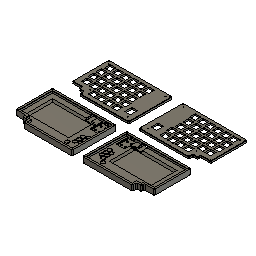
Split_Keyboardd (Autodesk Fusion 360 design; units mm, degrees)
part number: 2026-06-04-13-11-55-782
Autodesk Fusion 360 part; units mm, degrees
note: some values were not read from the file. Chosen so that the rebuilt part matches the saved one: which bodies a step acts on; which pieces of a blend or face edit are solid. Set by a fixed rule: which sketch regions a step uses; the direction of a hole.
(part 1 of 2)
sketch "Sketch1" plane through (0, 0, 0) normal (0, 1, 0) x (1, 0, 0)
  line L0 (174.75, 46) -> (174.75, -34.5)
  line L1 (174.75, -34.5) -> (149.75, -34.5)
  line L2 (149.75, -34.5) -> (149.75, -42)
  line L3 (149.75, -42) -> (138.25, -42)
  line L4 (138.25, -42) -> (138.25, -52.5)
  line L5 (138.25, -52.5) -> (24.5, -52.5)
  line L6 (25.5, 46) -> (24.5, -52.5)
  line L7 (-11.6355, 46.5) -> (-159.1355, 46.5)
  line L8 (-159.1355, 46.5) -> (-159.1355, -34)
  line L9 (-159.1355, -34) -> (-134.6355, -34)
  line L10 (-134.6355, -34) -> (-134.6355, -41.5)
  line L11 (-134.6355, -41.5) -> (-123.1355, -41.5)
  line L12 (-123.1355, -41.5) -> (-123.1355, -52)
  line L13 (-123.1355, -52) -> (-11.6355, -52)
  line L14 (-11.6355, -52) -> (-11.6355, 46.5)
  line L15 (174.75, 46) -> (25.5, 46)
  line L16 (-164.1355, 49.5) -> (-164.1355, -37)
  line L17 (-162.1355, -39) -> (-141.6355, -39)
  line L18 (-139.6355, -41) -> (-139.6355, -44.5)
  line L19 (-137.6355, -46.5) -> (-130.1355, -46.5)
  line L20 (-128.1355, -48.5) -> (-128.1355, -55)
  line L21 (-126.1355, -57) -> (-8.6355, -57)
  line L22 (-6.6355, -55) -> (-6.6355, 49.5)
  line L23 (-8.6355, 51.5) -> (-162.1355, 51.5)
  line L24 (141.25, -57.5) -> (21.4694, -57.5)
  line L25 (20.5304, 49.0203) -> (19.4695, -55.4797)
  line L26 (177.75, 51) -> (22.5303, 51)
  line L27 (179.75, 49) -> (179.75, -37.5)
  line L28 (177.75, -39.5) -> (156.75, -39.5)
  line L29 (154.75, -41.5) -> (154.75, -45)
  line L30 (152.75, -47) -> (145.25, -47)
  line L31 (143.25, -49) -> (143.25, -55.5)
  line L32 (-159.1355, 46.5) -> (-145.2355, 46.5)
  line L33 (-145.2855, 36.0001) -> (-138.2355, 36)
  line L34 (-138.2355, 36) -> (-138.2356, 29)
  line L35 (-138.7356, 29) -> (-151.8356, 29)
  line L36 (-152.3356, 29.5) -> (-152.3356, 42.6)
  line L37 (-151.8356, 43.1) -> (-138.7356, 43.1)
  line L38 (-138.2356, 42.6) -> (-138.2356, 29.5)
  line L39 (-119.1356, 42.6) -> (-119.1356, 29.5)
  line L40 (-119.6356, 29) -> (-132.7356, 29)
  line L41 (-133.2356, 29.5) -> (-133.2356, 42.6)
  line L42 (-132.7356, 43.1) -> (-119.6356, 43.1)
  line L43 (-100.0356, 42.6) -> (-100.0356, 29.5)
  line L44 (-100.5356, 29) -> (-113.6356, 29)
  line L45 (-114.1356, 29.5) -> (-114.1356, 42.6)
  line L46 (-113.6356, 43.1) -> (-100.5356, 43.1)
  line L47 (-80.9356, 42.6) -> (-80.9356, 29.5)
  line L48 (-81.4356, 29) -> (-94.5356, 29)
  line L49 (-95.0356, 29.5) -> (-95.0356, 42.6)
  line L50 (-94.5356, 43.1) -> (-81.4356, 43.1)
  line L51 (-61.8356, 42.6) -> (-61.8356, 29.5)
  line L52 (-62.3356, 29) -> (-75.4356, 29)
  line L53 (-75.9356, 29.5) -> (-75.9356, 42.6)
  line L54 (-75.4356, 43.1) -> (-62.3356, 43.1)
  line L55 (-42.7356, 42.6) -> (-42.7356, 29.5)
  line L56 (-43.2356, 29) -> (-56.3356, 29)
  line L57 (-56.8356, 29.5) -> (-56.8356, 42.6)
  line L58 (-56.3356, 43.1) -> (-43.2356, 43.1)
  line L59 (-59.4356, 10.4) -> (-59.4356, 23.5)
  line L60 (-135.8356, 10.4) -> (-135.8356, 23.5)
  line L61 (-154.9356, 10.4) -> (-154.9356, 23.5)
  line L62 (-154.4356, 24) -> (-141.3356, 24)
  line L63 (-122.2356, 9.9) -> (-135.3356, 9.9)
  line L64 (-45.3356, 23.5) -> (-45.3356, 10.4)
  line L65 (-116.7356, 10.4) -> (-116.7356, 23.5)
  line L66 (-102.6356, 23.5) -> (-102.6356, 10.4)
  line L67 (-83.5356, 23.5) -> (-83.5356, 10.4)
  line L68 (-84.0356, 9.9) -> (-97.1356, 9.9)
  line L69 (-147.8855, 16.9001) -> (-140.8355, 16.9)
  line L70 (-141.3356, 9.9) -> (-154.4356, 9.9)
  line L71 (-140.8356, 23.5) -> (-140.8356, 9.9)
  line L72 (-78.5356, 10.4) -> (-78.5356, 23.5)
  line L73 (-121.7356, 23.5) -> (-121.7356, 10.4)
  line L74 (-135.3356, 24) -> (-122.2356, 24)
  line L75 (-140.8355, 16.9) -> (-140.8356, 10.4)
  line L76 (-103.1356, 9.9) -> (-116.2356, 9.9)
  line L77 (-78.0356, 24) -> (-64.9356, 24)
  line L78 (-97.6356, 10.4) -> (-97.6356, 23.5)
  line L79 (-116.2356, 24) -> (-103.1356, 24)
  line L80 (-97.1356, 24) -> (-84.0356, 24)
  line L81 (-45.8356, 9.9) -> (-58.9356, 9.9)
  line L82 (-64.9356, 9.9) -> (-78.0356, 9.9)
  line L83 (-64.4356, 23.5) -> (-64.4356, 10.4)
  line L84 (-58.9356, 24) -> (-45.8356, 24)
  line L85 (-135.8356, -8.7) -> (-135.8356, 4.4)
  line L86 (-78.0356, 4.9) -> (-64.9356, 4.9)
  line L87 (-83.5356, 4.4) -> (-83.5356, -8.7)
  line L88 (-84.0356, -9.2) -> (-97.1356, -9.2)
  line L89 (-45.3356, 4.4) -> (-45.3356, -8.7)
  line L90 (-58.9356, 4.9) -> (-45.8356, 4.9)
  line L91 (-154.4356, 4.9) -> (-141.3356, 4.9)
  line L92 (-154.9356, -8.7) -> (-154.9356, 4.4)
  line L93 (-59.4356, -8.7) -> (-59.4356, 4.4)
  line L94 (-45.8356, -9.2) -> (-58.9356, -9.2)
  line L95 (-78.5356, -8.7) -> (-78.5356, 4.4)
  line L96 (-97.1356, 4.9) -> (-84.0356, 4.9)
  line L97 (-97.6356, -8.7) -> (-97.6356, 4.4)
  line L98 (-121.7356, 4.4) -> (-121.7356, -8.7)
  line L99 (-140.8356, 4.4) -> (-140.8356, -9.2)
  line L100 (-64.4356, 4.4) -> (-64.4356, -8.7)
  line L101 (-64.9356, -9.2) -> (-78.0356, -9.2)
  line L102 (-103.1356, -9.2) -> (-116.2356, -9.2)
  line L103 (-116.2356, 4.9) -> (-103.1356, 4.9)
  line L104 (-122.2356, -9.2) -> (-135.3356, -9.2)
  line L105 (-102.6356, 4.4) -> (-102.6356, -8.7)
  line L106 (-140.8355, -2.2) -> (-140.8356, -8.7)
  line L107 (-116.7356, -8.7) -> (-116.7356, 4.4)
  line L108 (-147.8855, -2.1999) -> (-140.8355, -2.2)
  line L109 (-135.3356, 4.9) -> (-122.2356, 4.9)
  line L110 (-141.3356, -9.2) -> (-154.4356, -9.2)
  line L111 (-119.6356, -28.3) -> (-132.7356, -28.3)
  line L112 (-138.7356, -28.3) -> (-151.8356, -28.3)
  line L113 (-119.1356, -14.7) -> (-119.1356, -27.8)
  line L114 (-132.7356, -14.2) -> (-119.6356, -14.2)
  line L115 (-114.1356, -27.8) -> (-114.1356, -14.7)
  line L116 (-151.8356, -14.2) -> (-138.7356, -14.2)
  line L117 (-95.0356, -27.8) -> (-95.0356, -14.7)
  line L118 (-61.8356, -14.7) -> (-61.8356, -27.8)
  line L119 (-113.6356, -14.2) -> (-100.5356, -14.2)
  line L120 (-56.3356, -14.2) -> (-43.2356, -14.2)
  line L121 (-100.5356, -28.3) -> (-113.6356, -28.3)
  line L122 (-145.2855, -21.2999) -> (-138.2355, -21.3)
  line L123 (-75.4356, -14.2) -> (-62.3356, -14.2)
  line L124 (-81.4356, -28.3) -> (-94.5356, -28.3)
  line L125 (-43.2356, -28.3) -> (-56.3356, -28.3)
  line L126 (-100.0356, -14.7) -> (-100.0356, -27.8)
  line L127 (-94.5356, -14.2) -> (-81.4356, -14.2)
  line L128 (-138.2356, -14.7) -> (-138.2356, -28.3)
  line L129 (-152.3356, -27.8) -> (-152.3356, -14.7)
  line L130 (-138.2355, -21.3) -> (-138.2356, -27.8)
  line L131 (-75.9356, -27.8) -> (-75.9356, -14.7)
  line L132 (-133.2356, -27.8) -> (-133.2356, -14.7)
  line L133 (-80.9356, -14.7) -> (-80.9356, -27.8)
  line L134 (-42.7356, -14.7) -> (-42.7356, -27.8)
  line L135 (-56.8356, -27.8) -> (-56.8356, -14.7)
  line L136 (-62.3356, -28.3) -> (-75.4356, -28.3)
  line L137 (-102.6356, -33.8) -> (-102.6356, -46.9)
  line L138 (-116.7356, -46.9) -> (-116.7356, -33.8)
  line L139 (-83.5356, -33.8) -> (-83.5356, -46.9)
  line L140 (-58.9356, -33.3) -> (-45.8356, -33.3)
  line L141 (-97.1356, -33.3) -> (-85.0356, -33.3)
  line L142 (-97.6356, -46.9) -> (-97.6356, -33.8)
  line L143 (-103.1356, -47.4) -> (-116.2356, -47.4)
  line L144 (-64.4356, -33.8) -> (-64.4356, -46.9)
  line L145 (-45.8356, -47.4) -> (-58.9356, -47.4)
  line L146 (-116.2356, -33.3) -> (-103.1356, -33.3)
  line L147 (-78.0356, -33.3) -> (-64.9356, -33.3)
  line L148 (-84.0356, -47.4) -> (-97.1356, -47.4)
  line L149 (-45.3356, -33.8) -> (-45.3356, -46.9)
  line L150 (-64.9356, -47.4) -> (-78.0356, -47.4)
  line L151 (-59.4356, -46.9) -> (-59.4356, -33.8)
  line L152 (-78.5356, -46.9) -> (-78.5356, -33.8)
  line L153 (167.3, 28.95) -> (154.2, 28.95)
  line L154 (153.7, 29.45) -> (153.7, 42.55)
  line L155 (154.2, 43.05) -> (167.3, 43.05)
  line L156 (167.8, 42.55) -> (167.8, 29.45)
  line L157 (148.2, 28.95) -> (135.1, 28.95)
  line L158 (148.7, 42.55) -> (148.7, 29.45)
  line L159 (134.6, 29.45) -> (134.6, 42.55)
  line L160 (135.1, 43.05) -> (148.2, 43.05)
  line L161 (129.15, 28.95) -> (116.05, 28.95)
  line L162 (129.65, 42.55) -> (129.65, 29.45)
  line L163 (115.55, 29.45) -> (115.55, 42.55)
  line L164 (116.05, 43.05) -> (129.15, 43.05)
  line L165 (110.15, 28.95) -> (97.05, 28.95)
  line L166 (110.65, 42.55) -> (110.65, 29.45)
  line L167 (96.55, 29.45) -> (96.55, 42.55)
  line L168 (97.05, 43.05) -> (110.15, 43.05)
  line L169 (91.1, 28.95) -> (78, 28.95)
  line L170 (91.6, 42.55) -> (91.6, 29.45)
  line L171 (77.5, 29.45) -> (77.5, 42.55)
  line L172 (78, 43.05) -> (91.1, 43.05)
  line L173 (72.05, 28.95) -> (58.95, 28.95)
  line L174 (72.55, 42.55) -> (72.55, 29.45)
  line L175 (58.45, 29.45) -> (58.45, 42.55)
  line L176 (58.95, 43.05) -> (72.05, 43.05)
  line L177 (150.75, 9.9) -> (137.65, 9.9)
  line L178 (170.35, 23.5) -> (170.35, 10.4)
  line L179 (118.6, 24) -> (131.7, 24)
  line L180 (137.65, 24) -> (150.75, 24)
  line L181 (156.75, 24) -> (169.85, 24)
  line L182 (61, 10.4) -> (61, 23.5)
  line L183 (74.6, 9.9) -> (61.5, 9.9)
  line L184 (61.5, 24) -> (74.6, 24)
  line L185 (99.6, 24) -> (112.7, 24)
  line L186 (99.1, 10.4) -> (99.1, 23.5)
  line L187 (75.1, 23.5) -> (75.1, 10.4)
  line L188 (112.7, 9.9) -> (99.6, 9.9)
  line L189 (80.05, 10.4) -> (80.05, 23.5)
  line L190 (156.25, 10.4) -> (156.25, 23.5)
  line L191 (80.55, 24) -> (93.65, 24)
  line L192 (132.2, 23.5) -> (132.2, 10.4)
  line L193 (137.15, 10.4) -> (137.15, 23.5)
  line L194 (113.2, 23.5) -> (113.2, 10.4)
  line L195 (94.15, 23.5) -> (94.15, 10.4)
  line L196 (131.7, 9.9) -> (118.6, 9.9)
  line L197 (169.85, 9.9) -> (156.75, 9.9)
  line L198 (151.25, 23.5) -> (151.25, 10.4)
  line L199 (118.1, 10.4) -> (118.1, 23.5)
  line L200 (93.65, 9.9) -> (80.55, 9.9)
  line L201 (61, -8.65) -> (61, 4.45)
  line L202 (156.75, 4.95) -> (169.85, 4.95)
  line L203 (137.15, -8.65) -> (137.15, 4.45)
  line L204 (150.75, -9.15) -> (137.65, -9.15)
  line L205 (118.6, 4.95) -> (131.7, 4.95)
  line L206 (137.65, 4.95) -> (150.75, 4.95)
  line L207 (151.25, 4.45) -> (151.25, -8.65)
  line L208 (170.35, 4.45) -> (170.35, -8.65)
  line L209 (156.25, -8.65) -> (156.25, 4.45)
  line L210 (93.65, -9.15) -> (80.55, -9.15)
  line L211 (112.7, -9.15) -> (99.6, -9.15)
  line L212 (75.1, 4.45) -> (75.1, -8.65)
  line L213 (74.6, -9.15) -> (61.5, -9.15)
  line L214 (80.05, -8.65) -> (80.05, 4.45)
  line L215 (169.85, -9.15) -> (156.75, -9.15)
  line L216 (99.1, -8.65) -> (99.1, 4.45)
  line L217 (94.15, 4.45) -> (94.15, -8.65)
  line L218 (132.2, 4.45) -> (132.2, -8.65)
  line L219 (61.5, 4.95) -> (74.6, 4.95)
  line L220 (80.55, 4.95) -> (93.65, 4.95)
  line L221 (118.1, -8.65) -> (118.1, 4.45)
  line L222 (131.7, -9.15) -> (118.6, -9.15)
  line L223 (99.6, 4.95) -> (112.7, 4.95)
  line L224 (113.2, 4.45) -> (113.2, -8.65)
  line L225 (58.45, -27.7) -> (58.45, -14.6)
  line L226 (154.2, -14.1) -> (167.3, -14.1)
  line L227 (134.6, -27.7) -> (134.6, -14.6)
  line L228 (148.2, -28.2) -> (135.1, -28.2)
  line L229 (116.05, -14.1) -> (129.15, -14.1)
  line L230 (135.1, -14.1) -> (148.2, -14.1)
  line L231 (148.7, -14.6) -> (148.7, -27.7)
  line L232 (167.8, -14.6) -> (167.8, -27.7)
  line L233 (153.7, -27.7) -> (153.7, -14.6)
  line L234 (91.1, -28.2) -> (78, -28.2)
  line L235 (110.15, -28.2) -> (97.05, -28.2)
  line L236 (72.55, -14.6) -> (72.55, -27.7)
  line L237 (72.05, -28.2) -> (58.95, -28.2)
  line L238 (77.5, -27.7) -> (77.5, -14.6)
  line L239 (167.3, -28.2) -> (154.2, -28.2)
  line L240 (96.55, -27.7) -> (96.55, -14.6)
  line L241 (91.6, -14.6) -> (91.6, -27.7)
  line L242 (129.65, -14.6) -> (129.65, -27.7)
  line L243 (58.95, -14.1) -> (72.05, -14.1)
  line L244 (78, -14.1) -> (91.1, -14.1)
  line L245 (115.55, -27.7) -> (115.55, -14.6)
  line L246 (129.15, -28.2) -> (116.05, -28.2)
  line L247 (97.05, -14.1) -> (110.15, -14.1)
  line L248 (110.65, -14.6) -> (110.65, -27.7)
  line L249 (61, -46.75) -> (61, -33.65)
  line L250 (118.6, -33.15) -> (131.7, -33.15)
  line L251 (93.65, -47.25) -> (80.55, -47.25)
  line L252 (112.7, -47.25) -> (99.6, -47.25)
  line L253 (75.1, -33.65) -> (75.1, -46.75)
  line L254 (74.6, -47.25) -> (61.5, -47.25)
  line L255 (80.05, -46.75) -> (80.05, -33.65)
  line L256 (99.1, -46.75) -> (99.1, -33.65)
  line L257 (94.15, -33.65) -> (94.15, -46.75)
  line L258 (132.2, -33.65) -> (132.2, -46.75)
  line L259 (61.5, -33.15) -> (74.6, -33.15)
  line L260 (80.55, -33.15) -> (93.65, -33.15)
  line L261 (118.1, -46.75) -> (118.1, -33.65)
  line L262 (131.7, -47.25) -> (118.6, -47.25)
  line L263 (99.6, -33.15) -> (112.7, -33.15)
  line L264 (113.2, -33.65) -> (113.2, -46.75)
  line L265 (32.8996, -40.5802) -> (45.9015, -40.5802)
  line L266 (46.4015, -40.0802) -> (46.4015, -23.5802)
  line L267 (45.9015, -23.0802) -> (32.8996, -23.0802)
  line L268 (32.3996, -23.5802) -> (32.3996, -40.0802)
  line L269 (-11.6355, -52) -> (-19.6355, -52)
  line L270 (-20.1355, -39.5) -> (-33.1355, -39.5)
  line L271 (-33.6355, -39) -> (-33.6355, -22.5)
  line L272 (-33.1355, -22) -> (-20.1355, -22)
  line L273 (-19.6355, -22.5) -> (-19.6355, -39)
  arc A0 (19.4695, -55.4797) -> (21.4694, -57.5) centre (21.4694, -55.5) ccw
  arc A1 (141.25, -57.5) -> (143.25, -55.5) centre (141.25, -55.5) ccw
  arc A2 (145.25, -47) -> (143.25, -49) centre (145.25, -49) ccw
  arc A3 (152.75, -47) -> (154.75, -45) centre (152.75, -45) ccw
  arc A4 (156.75, -39.5) -> (154.75, -41.5) centre (156.75, -41.5) ccw
  arc A5 (177.75, -39.5) -> (179.75, -37.5) centre (177.75, -37.5) ccw
  arc A6 (179.75, 49) -> (177.75, 51) centre (177.75, 49) ccw
  arc A7 (22.5303, 51) -> (20.5304, 49.0203) centre (22.5303, 49) ccw
  arc A8 (-8.6355, -57) -> (-6.6355, -55) centre (-8.6355, -55) ccw
  arc A9 (-6.6355, 49.5) -> (-8.6355, 51.5) centre (-8.6355, 49.5) ccw
  arc A10 (-162.1355, 51.5) -> (-164.1355, 49.5) centre (-162.1355, 49.5) ccw
  arc A11 (-164.1355, -37) -> (-162.1355, -39) centre (-162.1355, -37) ccw
  arc A12 (-139.6355, -41) -> (-141.6355, -39) centre (-141.6355, -41) ccw
  arc A13 (-139.6355, -44.5) -> (-137.6355, -46.5) centre (-137.6355, -44.5) ccw
  arc A14 (-128.1355, -48.5) -> (-130.1355, -46.5) centre (-130.1355, -48.5) ccw
  arc A15 (-128.1355, -55) -> (-126.1355, -57) centre (-126.1355, -55) ccw
  arc A16 (-151.8356, 43.1) -> (-152.3356, 42.6) centre (-151.8356, 42.6) ccw
  arc A17 (-138.2356, 42.6) -> (-138.7356, 43.1) centre (-138.7356, 42.6) ccw
  arc A18 (-152.3356, 29.5) -> (-151.8356, 29) centre (-151.8356, 29.5) ccw
  arc A19 (-133.2356, 29.5) -> (-132.7356, 29) centre (-132.7356, 29.5) ccw
  arc A20 (-132.7356, 43.1) -> (-133.2356, 42.6) centre (-132.7356, 42.6) ccw
  arc A21 (-119.1356, 42.6) -> (-119.6356, 43.1) centre (-119.6356, 42.6) ccw
  arc A22 (-119.6356, 29) -> (-119.1356, 29.5) centre (-119.6356, 29.5) ccw
  arc A23 (-114.1356, 29.5) -> (-113.6356, 29) centre (-113.6356, 29.5) ccw
  arc A24 (-113.6356, 43.1) -> (-114.1356, 42.6) centre (-113.6356, 42.6) ccw
  arc A25 (-100.0356, 42.6) -> (-100.5356, 43.1) centre (-100.5356, 42.6) ccw
  arc A26 (-100.5356, 29) -> (-100.0356, 29.5) centre (-100.5356, 29.5) ccw
  arc A27 (-95.0356, 29.5) -> (-94.5356, 29) centre (-94.5356, 29.5) ccw
  arc A28 (-94.5356, 43.1) -> (-95.0356, 42.6) centre (-94.5356, 42.6) ccw
  arc A29 (-80.9356, 42.6) -> (-81.4356, 43.1) centre (-81.4356, 42.6) ccw
  arc A30 (-81.4356, 29) -> (-80.9356, 29.5) centre (-81.4356, 29.5) ccw
  arc A31 (-83.5356, 23.5) -> (-84.0356, 24) centre (-84.0356, 23.5) ccw
  arc A32 (-97.1356, 24) -> (-97.6356, 23.5) centre (-97.1356, 23.5) ccw
  arc A33 (-97.6356, 10.4) -> (-97.1356, 9.9) centre (-97.1356, 10.4) ccw
  arc A34 (-84.0356, 9.9) -> (-83.5356, 10.4) centre (-84.0356, 10.4) ccw
  arc A35 (-102.6356, 23.5) -> (-103.1356, 24) centre (-103.1356, 23.5) ccw
  arc A36 (-116.7356, 10.4) -> (-116.2356, 9.9) centre (-116.2356, 10.4) ccw
  arc A37 (-116.2356, 24) -> (-116.7356, 23.5) centre (-116.2356, 23.5) ccw
  arc A38 (-103.1356, 9.9) -> (-102.6356, 10.4) centre (-103.1356, 10.4) ccw
  arc A39 (-121.7356, 23.5) -> (-122.2356, 24) centre (-122.2356, 23.5) ccw
  arc A40 (-122.2356, 9.9) -> (-121.7356, 10.4) centre (-122.2356, 10.4) ccw
  arc A41 (-135.8356, 10.4) -> (-135.3356, 9.9) centre (-135.3356, 10.4) ccw
  arc A42 (-135.3356, 24) -> (-135.8356, 23.5) centre (-135.3356, 23.5) ccw
  arc A43 (-140.8356, 23.5) -> (-141.3356, 24) centre (-141.3356, 23.5) ccw
  arc A44 (-154.9356, 10.4) -> (-154.4356, 9.9) centre (-154.4356, 10.4) ccw
  arc A45 (-154.4356, 24) -> (-154.9356, 23.5) centre (-154.4356, 23.5) ccw
  arc A46 (-75.4356, 43.1) -> (-75.9356, 42.6) centre (-75.4356, 42.6) ccw
  arc A47 (-61.8356, 42.6) -> (-62.3356, 43.1) centre (-62.3356, 42.6) ccw
  arc A48 (-62.3356, 29) -> (-61.8356, 29.5) centre (-62.3356, 29.5) ccw
  arc A49 (-75.9356, 29.5) -> (-75.4356, 29) centre (-75.4356, 29.5) ccw
  arc A50 (-64.4356, 23.5) -> (-64.9356, 24) centre (-64.9356, 23.5) ccw
  arc A51 (-64.9356, 9.9) -> (-64.4356, 10.4) centre (-64.9356, 10.4) ccw
  arc A52 (-78.0356, 24) -> (-78.5356, 23.5) centre (-78.0356, 23.5) ccw
  arc A53 (-78.5356, 10.4) -> (-78.0356, 9.9) centre (-78.0356, 10.4) ccw
  arc A54 (-138.7356, 29) -> (-138.2356, 29.5) centre (-138.7356, 29.5) ccw
  arc A55 (-141.3356, 9.9) -> (-140.8356, 10.4) centre (-141.3356, 10.4) ccw
  arc A56 (-141.3356, -9.2) -> (-140.8356, -8.7) centre (-141.3356, -8.7) ccw
  arc A57 (-140.8356, 4.4) -> (-141.3356, 4.9) centre (-141.3356, 4.4) ccw
  arc A58 (-154.4356, 4.9) -> (-154.9356, 4.4) centre (-154.4356, 4.4) ccw
  arc A59 (-154.9356, -8.7) -> (-154.4356, -9.2) centre (-154.4356, -8.7) ccw
  arc A60 (-135.3356, 4.9) -> (-135.8356, 4.4) centre (-135.3356, 4.4) ccw
  arc A61 (-121.7356, 4.4) -> (-122.2356, 4.9) centre (-122.2356, 4.4) ccw
  arc A62 (-122.2356, -9.2) -> (-121.7356, -8.7) centre (-122.2356, -8.7) ccw
  arc A63 (-135.8356, -8.7) -> (-135.3356, -9.2) centre (-135.3356, -8.7) ccw
  arc A64 (-116.2356, 4.9) -> (-116.7356, 4.4) centre (-116.2356, 4.4) ccw
  arc A65 (-102.6356, 4.4) -> (-103.1356, 4.9) centre (-103.1356, 4.4) ccw
  arc A66 (-103.1356, -9.2) -> (-102.6356, -8.7) centre (-103.1356, -8.7) ccw
  arc A67 (-116.7356, -8.7) -> (-116.2356, -9.2) centre (-116.2356, -8.7) ccw
  arc A68 (-97.1356, 4.9) -> (-97.6356, 4.4) centre (-97.1356, 4.4) ccw
  arc A69 (-97.6356, -8.7) -> (-97.1356, -9.2) centre (-97.1356, -8.7) ccw
  arc A70 (-83.5356, 4.4) -> (-84.0356, 4.9) centre (-84.0356, 4.4) ccw
  arc A71 (-84.0356, -9.2) -> (-83.5356, -8.7) centre (-84.0356, -8.7) ccw
  arc A72 (-78.0356, 4.9) -> (-78.5356, 4.4) centre (-78.0356, 4.4) ccw
  arc A73 (-78.5356, -8.7) -> (-78.0356, -9.2) centre (-78.0356, -8.7) ccw
  arc A74 (-64.4356, 4.4) -> (-64.9356, 4.9) centre (-64.9356, 4.4) ccw
  arc A75 (-64.9356, -9.2) -> (-64.4356, -8.7) centre (-64.9356, -8.7) ccw
  arc A76 (-58.9356, 4.9) -> (-59.4356, 4.4) centre (-58.9356, 4.4) ccw
  arc A77 (-59.4356, -8.7) -> (-58.9356, -9.2) centre (-58.9356, -8.7) ccw
  arc A78 (-45.3356, 4.4) -> (-45.8356, 4.9) centre (-45.8356, 4.4) ccw
  arc A79 (-45.8356, -9.2) -> (-45.3356, -8.7) centre (-45.8356, -8.7) ccw
  arc A80 (-45.8356, 9.9) -> (-45.3356, 10.4) centre (-45.8356, 10.4) ccw
  arc A81 (-59.4356, 10.4) -> (-58.9356, 9.9) centre (-58.9356, 10.4) ccw
  arc A82 (-58.9356, 24) -> (-59.4356, 23.5) centre (-58.9356, 23.5) ccw
  arc A83 (-45.3356, 23.5) -> (-45.8356, 24) centre (-45.8356, 23.5) ccw
  arc A84 (-43.2356, 29) -> (-42.7356, 29.5) centre (-43.2356, 29.5) ccw
  arc A85 (-56.8356, 29.5) -> (-56.3356, 29) centre (-56.3356, 29.5) ccw
  arc A86 (-56.3356, 43.1) -> (-56.8356, 42.6) centre (-56.3356, 42.6) ccw
  arc A87 (-42.7356, 42.6) -> (-43.2356, 43.1) centre (-43.2356, 42.6) ccw
  arc A88 (-138.2356, -14.7) -> (-138.7356, -14.2) centre (-138.7356, -14.7) ccw
  arc A89 (-151.8356, -14.2) -> (-152.3356, -14.7) centre (-151.8356, -14.7) ccw
  arc A90 (-152.3356, -27.8) -> (-151.8356, -28.3) centre (-151.8356, -27.8) ccw
  arc A91 (-132.7356, -14.2) -> (-133.2356, -14.7) centre (-132.7356, -14.7) ccw
  arc A92 (-133.2356, -27.8) -> (-132.7356, -28.3) centre (-132.7356, -27.8) ccw
  arc A93 (-119.1356, -14.7) -> (-119.6356, -14.2) centre (-119.6356, -14.7) ccw
  arc A94 (-119.6356, -28.3) -> (-119.1356, -27.8) centre (-119.6356, -27.8) ccw
  arc A95 (-116.2356, -33.3) -> (-116.7356, -33.8) centre (-116.2356, -33.8) ccw
  arc A96 (-116.7356, -46.9) -> (-116.2356, -47.4) centre (-116.2356, -46.9) ccw
  arc A97 (-102.6356, -33.8) -> (-103.1356, -33.3) centre (-103.1356, -33.8) ccw
  arc A98 (-103.1356, -47.4) -> (-102.6356, -46.9) centre (-103.1356, -46.9) ccw
  arc A99 (-100.5356, -28.3) -> (-100.0356, -27.8) centre (-100.5356, -27.8) ccw
  arc A100 (-100.0356, -14.7) -> (-100.5356, -14.2) centre (-100.5356, -14.7) ccw
  arc A101 (-113.6356, -14.2) -> (-114.1356, -14.7) centre (-113.6356, -14.7) ccw
  arc A102 (-114.1356, -27.8) -> (-113.6356, -28.3) centre (-113.6356, -27.8) ccw
  arc A103 (-94.5356, -14.2) -> (-95.0356, -14.7) centre (-94.5356, -14.7) ccw
  arc A104 (-80.9356, -14.7) -> (-81.4356, -14.2) centre (-81.4356, -14.7) ccw
  arc A105 (-75.4356, -14.2) -> (-75.9356, -14.7) centre (-75.4356, -14.7) ccw
  arc A106 (-61.8356, -14.7) -> (-62.3356, -14.2) centre (-62.3356, -14.7) ccw
  arc A107 (-56.3356, -14.2) -> (-56.8356, -14.7) centre (-56.3356, -14.7) ccw
  arc A108 (-42.7356, -14.7) -> (-43.2356, -14.2) centre (-43.2356, -14.7) ccw
  arc A109 (-43.2356, -28.3) -> (-42.7356, -27.8) centre (-43.2356, -27.8) ccw
  arc A110 (-56.8356, -27.8) -> (-56.3356, -28.3) centre (-56.3356, -27.8) ccw
  arc A111 (-62.3356, -28.3) -> (-61.8356, -27.8) centre (-62.3356, -27.8) ccw
  arc A112 (-75.9356, -27.8) -> (-75.4356, -28.3) centre (-75.4356, -27.8) ccw
  arc A113 (-81.4356, -28.3) -> (-80.9356, -27.8) centre (-81.4356, -27.8) ccw
  arc A114 (-95.0356, -27.8) -> (-94.5356, -28.3) centre (-94.5356, -27.8) ccw
  arc A115 (-83.5356, -33.8) -> (-84.5356, -33.8) centre (-84.0356, -33.8) ccw
  arc A116 (-97.1356, -33.3) -> (-97.6356, -33.8) centre (-97.1356, -33.8) ccw
  arc A117 (-97.6356, -46.9) -> (-97.1356, -47.4) centre (-97.1356, -46.9) ccw
  arc A118 (-84.5356, -33.8) -> (-85.0356, -33.3) centre (-85.0356, -33.8) ccw
  arc A119 (-84.0356, -47.4) -> (-83.5356, -46.9) centre (-84.0356, -46.9) ccw
  arc A120 (-78.0356, -33.3) -> (-78.5356, -33.8) centre (-78.0356, -33.8) ccw
  arc A121 (-78.5356, -46.9) -> (-78.0356, -47.4) centre (-78.0356, -46.9) ccw
  arc A122 (-64.4356, -33.8) -> (-64.9356, -33.3) centre (-64.9356, -33.8) ccw
  arc A123 (-64.9356, -47.4) -> (-64.4356, -46.9) centre (-64.9356, -46.9) ccw
  arc A124 (-58.9356, -33.3) -> (-59.4356, -33.8) centre (-58.9356, -33.8) ccw
  arc A125 (-59.4356, -46.9) -> (-58.9356, -47.4) centre (-58.9356, -46.9) ccw
  arc A126 (-45.3356, -33.8) -> (-45.8356, -33.3) centre (-45.8356, -33.8) ccw
  arc A127 (-45.8356, -47.4) -> (-45.3356, -46.9) centre (-45.8356, -46.9) ccw
  arc A128 (-33.1355, -22) -> (-33.6355, -22.5) centre (-33.1355, -22.5) ccw
  arc A129 (-19.6355, -22.5) -> (-20.1355, -22) centre (-20.1355, -22.5) ccw
  arc A130 (-20.1355, -39.5) -> (-19.6355, -39) centre (-20.1355, -39) ccw
  arc A131 (-33.6355, -39) -> (-33.1355, -39.5) centre (-33.1355, -39) ccw
  arc A132 (-138.7356, -28.3) -> (-138.2356, -27.8) centre (-138.7356, -27.8) ccw
  arc A133 (32.8996, -23.0802) -> (32.3996, -23.5802) centre (32.8996, -23.5802) ccw
  arc A134 (46.4015, -23.5802) -> (45.9015, -23.0802) centre (45.9015, -23.5802) ccw
  arc A135 (45.9015, -40.5802) -> (46.4015, -40.0802) centre (45.9015, -40.0802) ccw
  arc A136 (32.3996, -40.0802) -> (32.8996, -40.5802) centre (32.8996, -40.0802) ccw
  arc A137 (61.5, -33.15) -> (61, -33.65) centre (61.5, -33.65) ccw
  arc A138 (75.1, -33.65) -> (74.6, -33.15) centre (74.6, -33.65) ccw
  arc A139 (74.6, -47.25) -> (75.1, -46.75) centre (74.6, -46.75) ccw
  arc A140 (61, -46.75) -> (61.5, -47.25) centre (61.5, -46.75) ccw
  arc A141 (80.55, -33.15) -> (80.05, -33.65) centre (80.55, -33.65) ccw
  arc A142 (94.15, -33.65) -> (93.65, -33.15) centre (93.65, -33.65) ccw
  arc A143 (93.65, -47.25) -> (94.15, -46.75) centre (93.65, -46.75) ccw
  arc A144 (80.05, -46.75) -> (80.55, -47.25) centre (80.55, -46.75) ccw
  arc A145 (99.6, -33.15) -> (99.1, -33.65) centre (99.6, -33.65) ccw
  arc A146 (113.2, -33.65) -> (112.7, -33.15) centre (112.7, -33.65) ccw
  arc A147 (112.7, -47.25) -> (113.2, -46.75) centre (112.7, -46.75) ccw
  arc A148 (99.1, -46.75) -> (99.6, -47.25) centre (99.6, -46.75) ccw
  arc A149 (118.6, -33.15) -> (118.1, -33.65) centre (118.6, -33.65) ccw
  arc A150 (118.1, -46.75) -> (118.6, -47.25) centre (118.6, -46.75) ccw
  arc A151 (132.2, -33.65) -> (131.7, -33.15) centre (131.7, -33.65) ccw
  arc A152 (131.7, -47.25) -> (132.2, -46.75) centre (131.7, -46.75) ccw
  arc A153 (129.15, -28.2) -> (129.65, -27.7) centre (129.15, -27.7) ccw
  arc A154 (129.65, -14.6) -> (129.15, -14.1) centre (129.15, -14.6) ccw
  arc A155 (116.05, -14.1) -> (115.55, -14.6) centre (116.05, -14.6) ccw
  arc A156 (115.55, -27.7) -> (116.05, -28.2) centre (116.05, -27.7) ccw
  arc A157 (110.15, -28.2) -> (110.65, -27.7) centre (110.15, -27.7) ccw
  arc A158 (110.65, -14.6) -> (110.15, -14.1) centre (110.15, -14.6) ccw
  arc A159 (97.05, -14.1) -> (96.55, -14.6) centre (97.05, -14.6) ccw
  arc A160 (96.55, -27.7) -> (97.05, -28.2) centre (97.05, -27.7) ccw
  arc A161 (91.6, -14.6) -> (91.1, -14.1) centre (91.1, -14.6) ccw
  arc A162 (91.1, -28.2) -> (91.6, -27.7) centre (91.1, -27.7) ccw
  arc A163 (78, -14.1) -> (77.5, -14.6) centre (78, -14.6) ccw
  arc A164 (77.5, -27.7) -> (78, -28.2) centre (78, -27.7) ccw
  arc A165 (72.55, -14.6) -> (72.05, -14.1) centre (72.05, -14.6) ccw
  arc A166 (72.05, -28.2) -> (72.55, -27.7) centre (72.05, -27.7) ccw
  arc A167 (58.95, -14.1) -> (58.45, -14.6) centre (58.95, -14.6) ccw
  arc A168 (58.45, -27.7) -> (58.95, -28.2) centre (58.95, -27.7) ccw
  arc A169 (61.5, 4.95) -> (61, 4.45) centre (61.5, 4.45) ccw
  arc A170 (61, -8.65) -> (61.5, -9.15) centre (61.5, -8.65) ccw
  arc A171 (75.1, 4.45) -> (74.6, 4.95) centre (74.6, 4.45) ccw
  arc A172 (74.6, -9.15) -> (75.1, -8.65) centre (74.6, -8.65) ccw
  arc A173 (80.55, 4.95) -> (80.05, 4.45) centre (80.55, 4.45) ccw
  arc A174 (80.05, -8.65) -> (80.55, -9.15) centre (80.55, -8.65) ccw
  arc A175 (94.15, 4.45) -> (93.65, 4.95) centre (93.65, 4.45) ccw
  arc A176 (93.65, -9.15) -> (94.15, -8.65) centre (93.65, -8.65) ccw
  arc A177 (99.6, 4.95) -> (99.1, 4.45) centre (99.6, 4.45) ccw
  arc A178 (99.1, -8.65) -> (99.6, -9.15) centre (99.6, -8.65) ccw
  arc A179 (113.2, 4.45) -> (112.7, 4.95) centre (112.7, 4.45) ccw
  arc A180 (112.7, -9.15) -> (113.2, -8.65) centre (112.7, -8.65) ccw
  arc A181 (118.6, 4.95) -> (118.1, 4.45) centre (118.6, 4.45) ccw
  arc A182 (118.1, -8.65) -> (118.6, -9.15) centre (118.6, -8.65) ccw
  arc A183 (132.2, 4.45) -> (131.7, 4.95) centre (131.7, 4.45) ccw
  arc A184 (131.7, -9.15) -> (132.2, -8.65) centre (131.7, -8.65) ccw
  arc A185 (135.1, -14.1) -> (134.6, -14.6) centre (135.1, -14.6) ccw
  arc A186 (134.6, -27.7) -> (135.1, -28.2) centre (135.1, -27.7) ccw
  arc A187 (148.7, -14.6) -> (148.2, -14.1) centre (148.2, -14.6) ccw
  arc A188 (148.2, -28.2) -> (148.7, -27.7) centre (148.2, -27.7) ccw
  arc A189 (154.2, -14.1) -> (153.7, -14.6) centre (154.2, -14.6) ccw
  arc A190 (153.7, -27.7) -> (154.2, -28.2) centre (154.2, -27.7) ccw
  arc A191 (167.8, -14.6) -> (167.3, -14.1) centre (167.3, -14.6) ccw
  arc A192 (167.3, -28.2) -> (167.8, -27.7) centre (167.3, -27.7) ccw
  arc A193 (137.65, 4.95) -> (137.15, 4.45) centre (137.65, 4.45) ccw
  arc A194 (151.25, 4.45) -> (150.75, 4.95) centre (150.75, 4.45) ccw
  arc A195 (150.75, -9.15) -> (151.25, -8.65) centre (150.75, -8.65) ccw
  arc A196 (137.15, -8.65) -> (137.65, -9.15) centre (137.65, -8.65) ccw
  arc A197 (156.75, 4.95) -> (156.25, 4.45) centre (156.75, 4.45) ccw
  arc A198 (170.35, 4.45) -> (169.85, 4.95) centre (169.85, 4.45) ccw
  arc A199 (169.85, -9.15) -> (170.35, -8.65) centre (169.85, -8.65) ccw
  arc A200 (156.25, -8.65) -> (156.75, -9.15) centre (156.75, -8.65) ccw
  arc A201 (156.75, 24) -> (156.25, 23.5) centre (156.75, 23.5) ccw
  arc A202 (156.25, 10.4) -> (156.75, 9.9) centre (156.75, 10.4) ccw
  arc A203 (170.35, 23.5) -> (169.85, 24) centre (169.85, 23.5) ccw
  arc A204 (169.85, 9.9) -> (170.35, 10.4) centre (169.85, 10.4) ccw
  arc A205 (150.75, 9.9) -> (151.25, 10.4) centre (150.75, 10.4) ccw
  arc A206 (151.25, 23.5) -> (150.75, 24) centre (150.75, 23.5) ccw
  arc A207 (137.65, 24) -> (137.15, 23.5) centre (137.65, 23.5) ccw
  arc A208 (137.15, 10.4) -> (137.65, 9.9) centre (137.65, 10.4) ccw
  arc A209 (131.7, 9.9) -> (132.2, 10.4) centre (131.7, 10.4) ccw
  arc A210 (132.2, 23.5) -> (131.7, 24) centre (131.7, 23.5) ccw
  arc A211 (118.6, 24) -> (118.1, 23.5) centre (118.6, 23.5) ccw
  arc A212 (118.1, 10.4) -> (118.6, 9.9) centre (118.6, 10.4) ccw
  arc A213 (113.2, 23.5) -> (112.7, 24) centre (112.7, 23.5) ccw
  arc A214 (99.6, 24) -> (99.1, 23.5) centre (99.6, 23.5) ccw
  arc A215 (99.1, 10.4) -> (99.6, 9.9) centre (99.6, 10.4) ccw
  arc A216 (112.7, 9.9) -> (113.2, 10.4) centre (112.7, 10.4) ccw
  arc A217 (110.65, 42.55) -> (110.15, 43.05) centre (110.15, 42.55) ccw
  arc A218 (97.05, 43.05) -> (96.55, 42.55) centre (97.05, 42.55) ccw
  arc A219 (96.55, 29.45) -> (97.05, 28.95) centre (97.05, 29.45) ccw
  arc A220 (110.15, 28.95) -> (110.65, 29.45) centre (110.15, 29.45) ccw
  arc A221 (116.05, 43.05) -> (115.55, 42.55) centre (116.05, 42.55) ccw
  arc A222 (115.55, 29.45) -> (116.05, 28.95) centre (116.05, 29.45) ccw
  arc A223 (129.65, 42.55) -> (129.15, 43.05) centre (129.15, 42.55) ccw
  arc A224 (129.15, 28.95) -> (129.65, 29.45) centre (129.15, 29.45) ccw
  arc A225 (135.1, 43.05) -> (134.6, 42.55) centre (135.1, 42.55) ccw
  arc A226 (134.6, 29.45) -> (135.1, 28.95) centre (135.1, 29.45) ccw
  arc A227 (148.7, 42.55) -> (148.2, 43.05) centre (148.2, 42.55) ccw
  arc A228 (148.2, 28.95) -> (148.7, 29.45) centre (148.2, 29.45) ccw
  arc A229 (154.2, 43.05) -> (153.7, 42.55) centre (154.2, 42.55) ccw
  arc A230 (153.7, 29.45) -> (154.2, 28.95) centre (154.2, 29.45) ccw
  arc A231 (167.8, 42.55) -> (167.3, 43.05) centre (167.3, 42.55) ccw
  arc A232 (167.3, 28.95) -> (167.8, 29.45) centre (167.3, 29.45) ccw
  arc A233 (91.6, 42.55) -> (91.1, 43.05) centre (91.1, 42.55) ccw
  arc A234 (78, 43.05) -> (77.5, 42.55) centre (78, 42.55) ccw
  arc A235 (77.5, 29.45) -> (78, 28.95) centre (78, 29.45) ccw
  arc A236 (91.1, 28.95) -> (91.6, 29.45) centre (91.1, 29.45) ccw
  arc A237 (72.05, 28.95) -> (72.55, 29.45) centre (72.05, 29.45) ccw
  arc A238 (72.55, 42.55) -> (72.05, 43.05) centre (72.05, 42.55) ccw
  arc A239 (58.95, 43.05) -> (58.45, 42.55) centre (58.95, 42.55) ccw
  arc A240 (58.45, 29.45) -> (58.95, 28.95) centre (58.95, 29.45) ccw
  arc A241 (75.1, 23.5) -> (74.6, 24) centre (74.6, 23.5) ccw
  arc A242 (61.5, 24) -> (61, 23.5) centre (61.5, 23.5) ccw
  arc A243 (61, 10.4) -> (61.5, 9.9) centre (61.5, 10.4) ccw
  arc A244 (74.6, 9.9) -> (75.1, 10.4) centre (74.6, 10.4) ccw
  arc A245 (80.05, 10.4) -> (80.55, 9.9) centre (80.55, 10.4) ccw
  arc A246 (80.55, 24) -> (80.05, 23.5) centre (80.55, 23.5) ccw
  arc A247 (94.15, 23.5) -> (93.65, 24) centre (93.65, 23.5) ccw
  arc A248 (93.65, 9.9) -> (94.15, 10.4) centre (93.65, 10.4) ccw
  point P0 (170.75, 42)
  point P1 (29.5, 43)
  point P2 (31.9999, -47.1754)
  point P3 (140.2499, -35.0254)
  point P4 (-15.3855, 43.25)
  point P5 (-155.1355, 42)
  point P6 (-18.6355, -47)
  point P7 (-9.1355, 49)
  point P8 (-161.6355, 49)
  point P9 (-161.6355, -36.5)
  point P10 (-125.6355, -54.5)
  point P11 (-9.1355, -54.5)
  point P12 (23.0255, 48.5253)
  point P13 (177.25, 48.5)
  point P14 (177.25, -37)
  point P15 (140.75, -55)
  point P16 (22, -55)
  point P17 (32.3996, -40.5802)
  point P18 (32.3996, -23.0802)
  point P19 (-19.6355, -39.5)
  point P20 (-33.6355, -39.5)
  point P21 (-19.6355, -22)
  point P22 (-123.1355, -35.5)
  dimension "d1" = 149.25
  dimension "d2" = 80.5
  dimension "d3" = 25
  dimension "d7" = 113.75
  dimension "d11" = 147.5
  dimension "d12" = 80.5
  dimension "d13" = 24.5
  dimension "d15" = 11.5
  dimension "d18" = 111.5
  dimension "d87" = 17.5
  dimension "d90" = 8
  dimension "d92" = 17.5
  dimension "d93" = 14
  dimension "d94" = 2
  dimension "d95" = 0.5
  dimension "d96" = 0.5
  dimension "d97" = 0.5
  dimension "d98" = 0.5
  dimension "d99" = 0.5
  dimension "d100" = 0.5
  dimension "d105" = 6
  constraint perpendicular L0 L1
  constraint perpendicular L1 L2
  constraint perpendicular L2 L3
  constraint perpendicular L1 L4
  constraint perpendicular L4 L5
  constraint perpendicular L7 L8
  constraint perpendicular L8 L9
  constraint perpendicular L9 L10
  constraint perpendicular L10 L11
  constraint perpendicular L11 L12
  constraint perpendicular L12 L13
  constraint perpendicular L7 L14
  constraint horizontal L15
  constraint perpendicular L8 L32
  constraint perpendicular L33 L34
  constraint horizontal L35
  constraint vertical L36
  constraint horizontal L37
  constraint vertical L38
  constraint horizontal L40
  constraint vertical L41
  constraint horizontal L42
  constraint vertical L39
  constraint horizontal L44
  constraint vertical L45
  constraint horizontal L46
  constraint vertical L43
  constraint horizontal L48
  constraint vertical L49
  constraint horizontal L50
  constraint vertical L47
  constraint horizontal L52
  constraint vertical L53
  constraint horizontal L54
  constraint vertical L51
  constraint horizontal L56
  constraint vertical L57
  constraint horizontal L58
  constraint vertical L55
  constraint perpendicular L69 L75
  constraint horizontal L70
  constraint vertical L61
  constraint horizontal L62
  constraint vertical L71
  constraint horizontal L63
  constraint vertical L60
  constraint horizontal L74
  constraint vertical L73
  constraint horizontal L76
  constraint vertical L65
  constraint horizontal L79
  constraint vertical L66
  constraint horizontal L68
  constraint vertical L78
  constraint horizontal L80
  constraint vertical L67
  constraint horizontal L82
  constraint vertical L72
  constraint horizontal L77
  constraint vertical L83
  constraint horizontal L81
  constraint vertical L59
  constraint horizontal L84
  constraint vertical L64
  constraint perpendicular L106 L108
  constraint horizontal L110
  constraint vertical L92
  constraint horizontal L91
  constraint vertical L99
  constraint horizontal L104
  constraint vertical L85
  constraint horizontal L109
  constraint vertical L98
  constraint horizontal L102
  constraint vertical L107
  constraint horizontal L103
  constraint vertical L105
  constraint horizontal L88
  constraint vertical L97
  constraint horizontal L96
  constraint vertical L87
  constraint horizontal L101
  constraint vertical L95
  constraint horizontal L86
  constraint vertical L100
  constraint horizontal L94
  constraint vertical L93
  constraint horizontal L90
  constraint vertical L89
  constraint perpendicular L122 L130
  constraint horizontal L112
  constraint vertical L129
  constraint horizontal L116
  constraint vertical L128
  constraint horizontal L111
  constraint vertical L132
  constraint horizontal L114
  constraint vertical L113
  constraint horizontal L121
  constraint vertical L115
  constraint horizontal L119
  constraint vertical L126
  constraint horizontal L124
  constraint vertical L117
  constraint horizontal L127
  constraint vertical L133
  constraint horizontal L136
  constraint vertical L131
  constraint horizontal L123
  constraint vertical L118
  constraint horizontal L125
  constraint vertical L135
  constraint horizontal L120
  constraint vertical L134
  constraint horizontal L143
  constraint vertical L138
  constraint horizontal L146
  constraint vertical L137
  constraint horizontal L148
  constraint vertical L142
  constraint horizontal L141
  constraint vertical L139
  constraint horizontal L150
  constraint vertical L152
  constraint horizontal L147
  constraint vertical L144
  constraint horizontal L145
  constraint vertical L151
  constraint horizontal L140
  constraint vertical L149
  constraint horizontal L153
  constraint vertical L154
  constraint horizontal L155
  constraint perpendicular L153 L156
  constraint horizontal L157
  constraint vertical L159
  constraint horizontal L160
  constraint perpendicular L157 L158
  constraint horizontal L161
  constraint vertical L163
  constraint horizontal L164
  constraint perpendicular L161 L162
  constraint horizontal L165
  constraint vertical L167
  constraint horizontal L168
  constraint perpendicular L165 L166
  constraint horizontal L169
  constraint vertical L171
  constraint horizontal L172
  constraint perpendicular L169 L170
  constraint horizontal L173
  constraint vertical L175
  constraint horizontal L176
  constraint perpendicular L173 L174
  constraint horizontal L197
  constraint vertical L190
  constraint horizontal L181
  constraint perpendicular L178 L197
  constraint horizontal L177
  constraint vertical L193
  constraint horizontal L180
  constraint perpendicular L177 L198
  constraint horizontal L196
  constraint vertical L199
  constraint horizontal L179
  constraint perpendicular L192 L196
  constraint horizontal L188
  constraint vertical L186
  constraint horizontal L185
  constraint perpendicular L188 L194
  constraint horizontal L200
  constraint vertical L189
  constraint horizontal L191
  constraint perpendicular L195 L200
  constraint horizontal L183
  constraint vertical L182
  constraint horizontal L184
  constraint perpendicular L183 L187
  constraint horizontal L215
  constraint vertical L209
  constraint horizontal L202
  constraint perpendicular L208 L215
  constraint horizontal L204
  constraint vertical L203
  constraint horizontal L206
  constraint perpendicular L204 L207
  constraint horizontal L222
  constraint vertical L221
  constraint horizontal L205
  constraint perpendicular L218 L222
  constraint horizontal L211
  constraint vertical L216
  constraint horizontal L223
  constraint perpendicular L211 L224
  constraint horizontal L210
  constraint vertical L214
  constraint horizontal L220
  constraint perpendicular L210 L217
  constraint horizontal L213
  constraint vertical L201
  constraint horizontal L219
  constraint perpendicular L212 L213
  constraint horizontal L239
  constraint vertical L233
  constraint horizontal L226
  constraint perpendicular L232 L239
  constraint horizontal L228
  constraint vertical L227
  constraint horizontal L230
  constraint perpendicular L228 L231
  constraint horizontal L246
  constraint vertical L245
  constraint horizontal L229
  constraint perpendicular L242 L246
  constraint horizontal L235
  constraint vertical L240
  constraint horizontal L247
  constraint perpendicular L235 L248
  constraint horizontal L234
  constraint vertical L238
  constraint horizontal L244
  constraint perpendicular L234 L241
  constraint horizontal L237
  constraint vertical L225
  constraint horizontal L243
  constraint perpendicular L236 L237
  constraint horizontal L262
  constraint vertical L261
  constraint horizontal L250
  constraint perpendicular L258 L262
  constraint horizontal L252
  constraint vertical L256
  constraint horizontal L263
  constraint perpendicular L252 L264
  constraint horizontal L251
  constraint vertical L255
  constraint horizontal L260
  constraint perpendicular L251 L257
  constraint horizontal L254
  constraint vertical L249
  constraint horizontal L259
  constraint perpendicular L253 L254
  constraint horizontal L265
  constraint vertical L266
  constraint horizontal L267
  constraint vertical L268
  constraint perpendicular L14 L269
  constraint horizontal L270
  constraint vertical L271
  constraint horizontal L272
  constraint vertical L273
  constraint tangent L24 A0
  constraint tangent L25 A0
  constraint tangent L24 A1
  constraint tangent L31 A1
  constraint equal A0 A1
  constraint tangent L30 A2
  constraint tangent L31 A2
  constraint equal A0 A2
  constraint tangent L29 A3
  constraint tangent L30 A3
  constraint equal A0 A3
  constraint tangent L28 A4
  constraint tangent L29 A4
  constraint equal A0 A4
  constraint tangent L27 A5
  constraint tangent L28 A5
  constraint equal A0 A5
  constraint tangent L26 A6
  constraint tangent L27 A6
  constraint equal A0 A6
  constraint tangent L25 A7
  constraint tangent L26 A7
  constraint equal A0 A7
  constraint tangent L21 A8
  constraint tangent L22 A8
  constraint equal A0 A8
  constraint tangent L23 A9
  constraint tangent L22 A9
  constraint equal A0 A9
  constraint tangent L16 A10
  constraint tangent L23 A10
  constraint equal A0 A10
  constraint tangent L16 A11
  constraint tangent L17 A11
  constraint equal A0 A11
  constraint tangent L17 A12
  constraint tangent L18 A12
  constraint equal A0 A12
  constraint tangent L19 A13
  constraint tangent L18 A13
  constraint equal A0 A13
  constraint tangent L19 A14
  constraint tangent L20 A14
  constraint equal A0 A14
  constraint tangent L20 A15
  constraint tangent L21 A15
  constraint equal A0 A15
  constraint tangent L36 A16
  constraint tangent L37 A16
  constraint tangent L37 A17
  constraint tangent L38 A17
  constraint equal A16 A17
  constraint tangent L35 A18
  constraint tangent L36 A18
  constraint equal A16 A18
  constraint tangent L40 A19
  constraint tangent L41 A19
  constraint equal A16 A19
  constraint tangent L41 A20
  constraint tangent L42 A20
  constraint equal A16 A20
  constraint tangent L39 A21
  constraint tangent L42 A21
  constraint equal A16 A21
  constraint tangent L39 A22
  constraint tangent L40 A22
  constraint equal A16 A22
  constraint tangent L44 A23
  constraint tangent L45 A23
  constraint equal A16 A23
  constraint tangent L45 A24
  constraint tangent L46 A24
  constraint equal A16 A24
  constraint tangent L43 A25
  constraint tangent L46 A25
  constraint equal A16 A25
  constraint tangent L43 A26
  constraint tangent L44 A26
  constraint equal A16 A26
  constraint tangent L48 A27
  constraint tangent L49 A27
  constraint equal A16 A27
  constraint tangent L49 A28
  constraint tangent L50 A28
  constraint equal A16 A28
  constraint tangent L47 A29
  constraint tangent L50 A29
  constraint equal A16 A29
  constraint tangent L47 A30
  constraint tangent L48 A30
  constraint equal A16 A30
  constraint tangent L67 A31
  constraint tangent L80 A31
  constraint equal A16 A31
  constraint tangent L78 A32
  constraint tangent L80 A32
  constraint equal A16 A32
  constraint tangent L68 A33
  constraint tangent L78 A33
  constraint equal A16 A33
  constraint tangent L67 A34
  constraint tangent L68 A34
  constraint equal A16 A34
  constraint tangent L66 A35
  constraint tangent L79 A35
  constraint equal A16 A35
  constraint tangent L65 A36
  constraint tangent L76 A36
  constraint equal A16 A36
  constraint tangent L65 A37
  constraint tangent L79 A37
  constraint equal A16 A37
  constraint tangent L66 A38
  constraint tangent L76 A38
  constraint equal A16 A38
  constraint tangent L73 A39
  constraint tangent L74 A39
  constraint equal A16 A39
  constraint tangent L63 A40
  constraint tangent L73 A40
  constraint equal A16 A40
  constraint tangent L60 A41
  constraint tangent L63 A41
  constraint equal A16 A41
  constraint tangent L60 A42
  constraint tangent L74 A42
  constraint equal A16 A42
  constraint tangent L62 A43
  constraint tangent L71 A43
  constraint equal A16 A43
  constraint tangent L61 A44
  constraint tangent L70 A44
  constraint equal A16 A44
  constraint tangent L61 A45
  constraint tangent L62 A45
  constraint equal A16 A45
  constraint tangent L53 A46
  constraint tangent L54 A46
  constraint equal A16 A46
  constraint tangent L51 A47
  constraint tangent L54 A47
  constraint equal A16 A47
  constraint tangent L51 A48
  constraint tangent L52 A48
  constraint equal A16 A48
  constraint tangent L52 A49
  constraint tangent L53 A49
  constraint equal A16 A49
  constraint tangent L77 A50
  constraint tangent L83 A50
  constraint equal A16 A50
  constraint tangent L82 A51
  constraint tangent L83 A51
  constraint equal A16 A51
  constraint tangent L72 A52
  constraint tangent L77 A52
  constraint equal A16 A52
  constraint tangent L72 A53
  constraint tangent L82 A53
  constraint equal A16 A53
  constraint coincident L34.end L38
  constraint coincident L34.end L35
  constraint tangent L38 A54
  constraint tangent L35 A54
  constraint coincident L71.end L75
  constraint coincident L71.end L70
  constraint tangent L75 A55
  constraint tangent L70 A55
  constraint coincident L99.end L106
  constraint coincident L99.end L110
  constraint tangent L106 A56
  constraint tangent L110 A56
  constraint tangent L91 A57
  constraint tangent L99 A57
  constraint equal A56 A57
  constraint tangent L91 A58
  constraint tangent L92 A58
  constraint equal A56 A58
  constraint tangent L92 A59
  constraint tangent L110 A59
  constraint equal A56 A59
  constraint tangent L85 A60
  constraint tangent L109 A60
  constraint equal A56 A60
  constraint tangent L98 A61
  constraint tangent L109 A61
  constraint equal A56 A61
  constraint tangent L98 A62
  constraint tangent L104 A62
  constraint equal A56 A62
  constraint tangent L85 A63
  constraint tangent L104 A63
  constraint equal A56 A63
  constraint tangent L103 A64
  constraint tangent L107 A64
  constraint equal A56 A64
  constraint tangent L103 A65
  constraint tangent L105 A65
  constraint equal A56 A65
  constraint tangent L102 A66
  constraint tangent L105 A66
  constraint equal A56 A66
  constraint tangent L102 A67
  constraint tangent L107 A67
  constraint equal A56 A67
  constraint tangent L96 A68
  constraint tangent L97 A68
  constraint equal A56 A68
  constraint tangent L88 A69
  constraint tangent L97 A69
  constraint equal A56 A69
  constraint tangent L87 A70
  constraint tangent L96 A70
  constraint equal A56 A70
  constraint tangent L87 A71
  constraint tangent L88 A71
  constraint equal A56 A71
  constraint tangent L86 A72
  constraint tangent L95 A72
  constraint equal A56 A72
  constraint tangent L95 A73
  constraint tangent L101 A73
  constraint equal A56 A73
  constraint tangent L86 A74
  constraint tangent L100 A74
  constraint equal A56 A74
  constraint tangent L100 A75
  constraint tangent L101 A75
  constraint equal A56 A75
  constraint tangent L90 A76
  constraint tangent L93 A76
  constraint equal A56 A76
  constraint tangent L93 A77
  constraint tangent L94 A77
  constraint equal A56 A77
  constraint tangent L89 A78
  constraint tangent L90 A78
  constraint equal A56 A78
  constraint tangent L89 A79
  constraint tangent L94 A79
  constraint equal A56 A79
  constraint tangent L64 A80
  constraint tangent L81 A80
  constraint equal A56 A80
  constraint tangent L59 A81
  constraint tangent L81 A81
  constraint equal A56 A81
  constraint tangent L59 A82
  constraint tangent L84 A82
  constraint equal A56 A82
  constraint tangent L64 A83
  constraint tangent L84 A83
  constraint equal A56 A83
  constraint tangent L55 A84
  constraint tangent L56 A84
  constraint equal A56 A84
  constraint tangent L56 A85
  constraint tangent L57 A85
  constraint equal A56 A85
  constraint tangent L57 A86
  constraint tangent L58 A86
  constraint equal A56 A86
  constraint tangent L55 A87
  constraint tangent L58 A87
  constraint equal A56 A87
  constraint tangent L116 A88
  constraint tangent L128 A88
  constraint equal A56 A88
  constraint tangent L116 A89
  constraint tangent L129 A89
  constraint equal A56 A89
  constraint tangent L112 A90
  constraint tangent L129 A90
  constraint equal A56 A90
  constraint tangent L114 A91
  constraint tangent L132 A91
  constraint equal A56 A91
  constraint tangent L111 A92
  constraint tangent L132 A92
  constraint equal A56 A92
  constraint tangent L113 A93
  constraint tangent L114 A93
  constraint equal A56 A93
  constraint tangent L111 A94
  constraint tangent L113 A94
  constraint equal A56 A94
  constraint tangent L138 A95
  constraint tangent L146 A95
  constraint equal A56 A95
  constraint tangent L138 A96
  constraint tangent L143 A96
  constraint equal A56 A96
  constraint tangent L137 A97
  constraint tangent L146 A97
  constraint equal A56 A97
  constraint tangent L137 A98
  constraint tangent L143 A98
  constraint equal A56 A98
  constraint tangent L121 A99
  constraint tangent L126 A99
  constraint equal A56 A99
  constraint tangent L119 A100
  constraint tangent L126 A100
  constraint equal A56 A100
  constraint tangent L115 A101
  constraint tangent L119 A101
  constraint equal A56 A101
  constraint tangent L115 A102
  constraint tangent L121 A102
  constraint equal A56 A102
  constraint tangent L117 A103
  constraint tangent L127 A103
  constraint equal A56 A103
  constraint tangent L127 A104
  constraint tangent L133 A104
  constraint equal A56 A104
  constraint tangent L123 A105
  constraint tangent L131 A105
  constraint equal A56 A105
  constraint tangent L118 A106
  constraint tangent L123 A106
  constraint equal A56 A106
  constraint tangent L120 A107
  constraint tangent L135 A107
  constraint equal A56 A107
  constraint tangent L120 A108
  constraint tangent L134 A108
  constraint equal A56 A108
  constraint tangent L125 A109
  constraint tangent L134 A109
  constraint equal A56 A109
  constraint tangent L125 A110
  constraint tangent L135 A110
  constraint equal A56 A110